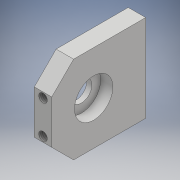
# Autodesk Inventor part: Base_roue
Saved by Autodesk Inventor 2018 (Build 220112000, 112)
## iProperties
Created: 2019-11-05
Part Number: Base_roue
Material: Generic
Document SubType Name: Modeling
Designer: hugo
Density: 1 g/cm^3
Appearance: Default
Author: hugo
Autodesk Inventor part; units mm, degrees
ref_plane "YZ Plane" through (0, 0, 0) normal (1, 0, 0) x (0, 1, 0)
ref_plane "XZ Plane" through (0, 0, 0) normal (0, 1, 0) x (-1, 0, 0)
ref_plane "XY Plane" through (0, 0, 0) normal (0, 0, 1) x (1, 0, 0)
sketch "Sketch1" plane through (0, 0, 0) normal (1, 0, 0) x (0, 1, 0)
  line L0 (12.5, 0) -> (53.8, 0)
  line L1 (53.8, 0) -> (53.8, -50)
  line L2 (53.8, -50) -> (12.5, -50)
  line L3 (0, -37.5) -> (0, -12.5)
  line L4 (0, -12.5) -> (12.5, 0)
  line L5 (53.8, -25) -> (0, -25) construction
  line L6 (0, -37.5) -> (12.5, -50)
  point P0 (0, 0)
  dimension "d1" = 50
  dimension "d2" = 12.5
  dimension "d3" = 45
  dimension "d4" = 53.8
  constraints: 14 end point, 2 midpoint, 2 parallel, 2 perpendicular, 2 symmetric about line, 1 horizontal
  measures "d1" distance of L0.end L1.end
  measures "d2" distance of L3.end point (0, 0)
  measures "d3" angle of L3 L4
  measures "d4" distance between parallel lines of L1 L3
extrude "Extrusion1" add sketch "Sketch1" along normal blind 10
sketch "Sketch2" plane through (10, 0, 0) normal (1, 0, 0) x (0, 0, -1)
  circle A0 centre (25, 24) radius 11
  line L0 (50, 53.8) -> (0, 53.8) projected
  line L1 (50, 12.5) -> (50, 53.8) projected
  point P0 (0, 0)
  dimension "d7" = 22
  dimension "d8" = 29.8
  dimension "d9" = 25
  constraints: 1 centre point
  measures "d7" diameter of A0
  measures "d8" distance from line of L0 A0.centre
  measures "d9" distance from line of L1 A0.centre
extrude "Extrusion2" cut sketch "Sketch2" against normal blind 7
sketch "Sketch3" plane through (3, 24, -25) normal (1, 0, 0) x (0, 0, -1)
  circle A0 centre (0, 0) radius 6
  point P0 (-25, -24)
  dimension "d12" = 12
  constraints: 1 centre point
  measures "d12" diameter of A0
extrude "Extrusion3" cut sketch "Sketch3" against normal blind 7
sketch "Sketch4" plane through (0, 53.8, 0) normal (0, 1, 0) x (1, 0, 0)
  line L0 (0, 19) -> (0, 31) construction
  line L1 (0, 25) -> (10, 25) construction
  line L2 (10, 12.5) -> (10, 37.5) construction
  line L3 (0, 0) -> (10, 0) construction
  line L4 (0, 50) -> (0, 0) construction
  point P0 (5, 10)
  point P1 (5, 40)
  dimension "d15" = 10
  dimension "d16" = 5
  constraints: 2 end point, 2 midpoint, 1 symmetric about line
  measures "d15" distance from line of L3 point (5, 10)
  measures "d16" distance from line of L4 point (5, 10)
hole "Hole1" at (5, 53.8, -10) at (5, 53.8, -40) direction (0, -1, 0) diameter 4.917 depth 28 tip angle 118 thread size "M6x1" class "6H" standard "ISO Metric profile"
sketch "Sketch5" plane through (0, 0, -37.5) normal (0, -1, 0) x (1, 0, 0)
  line L0 (10, 23.5) -> (10, 1.5) construction
  line L1 (10, 12.5) -> (0, 12.5) construction
  line L2 (0, 6.5) -> (0, 18.5) construction
  line L3 (0, 25) -> (10, 25) construction
  point P0 (0, 37.5)
  point P1 (5, 22)
  point P2 (5, 3)
  dimension "d24" = 5
  dimension "d25" = 3
  constraints: 2 end point, 2 midpoint, 1 symmetric about line
  measures "d24" distance from line of L0 point (5, 22)
  measures "d25" distance from line of L3 point (5, 22)
hole "Hole2" at (5, 0, -15.5) at (5, 0, -34.5) direction (0, 1, 0) diameter 4.917 depth 13 tip angle 118 thread size "M6x1" class "6H" standard "ISO Metric profile"
equation "\"d1\" = Hh"
equation "\"d2\" = 0.25 * Hh"
equation "\"d5\" = lR"
equation "\"d9\" = 0.5 * Hh"
equation "\"d16\" = 0.5 * lR"
equation "\"d24\" = 0.5 * lR"
equation "\"Hh\" = 50"
equation "\"lR\" = 10"
equation "\"Rr\" = 35"
equation "\"ha\" = 5"
equation "\"lp\" = 6"
equation "\"HR\" = -ha + Rr - lp"
equation "\"lr\" = 1.8"
body "Solid1"
